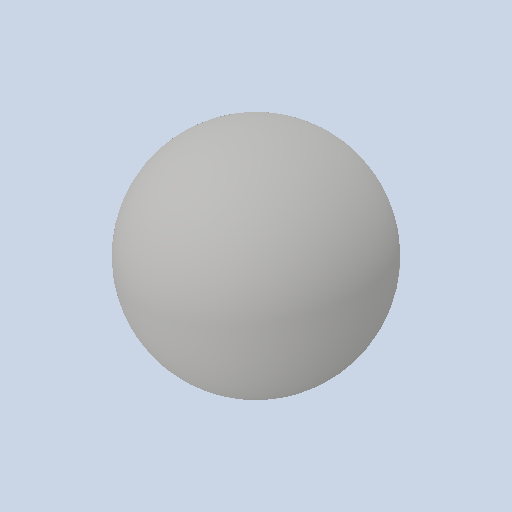
# Autodesk Inventor part: 040102DR-18-H8_ball_CPY
Saved by Autodesk Inventor 2024 (Build 280153000, 153)
## iProperties
Created: 2023-06-20
Part Number: 040102DR-18-H8_ball_CPY
Material: Generic
Catalog Web Link: www.cadenas.de
Description: DR-H ball-D-Series bearings
Vendor: TOKBEARING
Document SubType Name: Modeling
Designer: zegi
Manufacturer: TOKBEARING
Mass: 8700 g
Surface Area: 0.321699 cm^2
Volume: 0.0171573 cm^3
Density: 1 g/cm^3
Appearance: PSOLRGB-175-175-175
Category: PARTsolutions
Company: TOKBEARING
Title: 040102DR-18-H8_ball
Author: Cadenas PARTsolutions
Comments: D-Series bearings
PSOL_IDENT_0: {$CADENAS_DATA/23d-libs/tok_bearing/d_series_bearings/dr_h/dr_h_ball.prj},183 {VTYP=3D},{NB=040102DR
PSOL_IDENT_1: -18-H8_ball},{LINA=040102DR-18-H8_ball},{NN=DR-H ball},{DATE=16.12.2020 00:38:04},{GEOMDATE=19.02.20
PSOL_IDENT_2: 13 00:00:00},{VERSION=},{LINEID=1710},{WBVAR=},{WBNUMERIC=}  {NB=040102DR-18-H8_ball},{LINA=040102DR
PSOL_IDENT_3: -18-H8_ball},{KT=DUMMY},{IDNR=},{CODE=040102},{PN=DR-18-H8},{D=18},{SD=8.0},{W=5.0},{W1=-},{W1X=0.00
PSOL_IDENT_4: 0},{W2=-},{W2X=0.000},{LOAD=49 (5)},{TYPE=11},{QTY=3.000},{GW=8.7},{BD=3.2},{OP=42.704},{N=6},{R=6.8
PSOL_IDENT_5: },{GP=1.4}
NB: 040102DR-18-H8_ball
NN: DR-H ball
NT: D-Series bearings
NBSYN: $CODE.$PN._ball
LINA: 040102DR-18-H8_ball
CATALOG: TOK, Inc
CODE: 040102
PN: DR-18-H8
D: 18
SD: 8
W: 5
W1: -
W2: -
LOAD: 49 (5)
TYPE: 11
QTY: 3.000
GW: 8.7
SUPPLIER: TOKBEARING
ARTICLENO: 040102DR-18-H8_ball
BOMINFO: 040102DR-18-H8_ball
CREATOR: CADENAS GmbH
Autodesk Inventor part; units mm, degrees
sketch "Sketch_1" plane through (0, 0, 0) normal (0, 0, 1) x (1, 0, 0)
  line L0 (1.6, 0) -> (-1.6, 0)
  arc A0 (1.6, 0) -> (-1.6, 0) centre (0, 0) ccw
  line L1 (1.6, 0) -> (-1.6, 0)
  constraints: 4 end point, 2 point on circle, 1 centre point
revolve "Revolution1" add sketch "Sketch_1" angle 360 about axis through (1.6, 0, 0) along (1, 0, 0)
ref_plane "Ball_OR_XY" through (0, 0, 0) normal (1, 0, 0) x (0, 0, -1)
ref_plane "Ball_OR_YZ" through (0, 0, 0) normal (0, 0, -1) x (0, 1, 0)
ref_plane "Ball_OR_ZX" through (0, 0, 0) normal (0, 1, 0) x (1, 0, 0)
body "Solid1"
